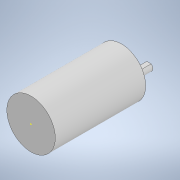
# Autodesk Inventor part: 29_Motore_6mm
Saved by Autodesk Inventor 2020.2 (Build 242310000, 310)
## iProperties
Created: 2020-01-17
Part Number: 29_Motore_6mm
Material: Generico
Document SubType Name: Modeling
Designer: socci
Density: 1 g/cm^3
Appearance: Default
Author: socci
Autodesk Inventor part; units mm, degrees
ref_plane "YZ Plane" through (0, 0, 0) normal (1, 0, 0) x (0, 1, 0)
ref_plane "XZ Plane" through (0, 0, 0) normal (0, 1, 0) x (-1, 0, 0)
ref_plane "XY Plane" through (0, 0, 0) normal (0, 0, 1) x (1, 0, 0)
sketch "Schizzo1" plane through (0, 0, 0) normal (0, 0, 1) x (1, 0, 0)
  circle A0 centre (0, 0) radius 18.5
  dimension "d0" = 37
  constraints: 1 centre point, 1 coincident
  measures "d0" diameter of A0
extrude "Estrusione1" add sketch "Schizzo1" along normal blind 69
sketch "Schizzo2" plane through (0, 0, 0) normal (0, 0, -1) x (-1, 0, 0)
  line L0 (0, 0) -> (15.3, 0)
  line L1 (0, 0) -> (15.3, 0) construction
  point P0 (7.65, 13.2502)
  point P1 (-7.65, 13.2502)
  point P2 (-15.3, 0)
  point P3 (-7.65, -13.2502)
  point P4 (7.65, -13.2502)
  dimension "d3" = 15.3
  dimension "d4" = 0
  dimension "d7" = 360
  constraints: 4 end point, 2 horizontal, 1 coincident, 1 collinear, 7 other
  measures "d3" distance of L0.start L0.end
  measures "d4" distance between parallel lines of L0 L1
hole "Foro1" at (7.65, 13.2502, 0) at (-7.65, 13.2502, 0) at (15.3, 0, 0) at (7.65, -13.2502, 0) at (-7.65, -13.2502, 0) at (-15.3, 0, 0) direction (0, 0, 1) diameter 2.459 depth 9 tip angle 118 thread size "M3x0.5" class "6H" standard "ISO Metric profile"
sketch "Schizzo3" plane through (0, 0, 0) normal (0, 0, -1) x (-1, 0, 0)
  circle A0 centre (0, 0) radius 18.5 projected
  line L0 (0, 18.5) -> (0, -0.9)
  line L1 (0, -0.9) -> (0, -6.9)
  circle A1 centre (0, -6.9) radius 6
  dimension "d16" = 19.4
  dimension "d17" = 6
  dimension "d18" = 12
  constraints: 4 end point, 1 centre point, 1 coincident, 1 point on line, 1 vertical, 1 vertical alignment, 1 other
  measures "d16" distance of L0.start L0.end
  measures "d17" distance of L0.end L1.end
  measures "d18" diameter of A1
extrude "Estrusione2" add sketch "Schizzo3" along normal blind 6 contours A1
sketch "Schizzo4" plane through (0, -6.9, -6) normal (0, 0, -1) x (-1, 0, 0)
  circle A0 centre (0, 0) radius 6 projected
  circle A1 centre (0, 0) radius 3
  point P0 (0, 6.9)
  dimension "d21" = 6
  constraints: 1 centre point, 1 coincident
  measures "d21" diameter of A1
extrude "Estrusione3" add sketch "Schizzo4" along normal blind 15 contours A1
sketch "Schizzo5" plane through (0, -6.9, -21) normal (0, 0, -1) x (-1, 0, 0)
  circle A0 centre (0, 0) radius 3
  circle A1 centre (0, 0) radius 3 projected
  line L0 (0, -3) -> (0, 2.5)
  line L1 (0, -3) -> (5.5, -3) construction
  line L2 (22.7528, -2.6034) -> (26.4877, -2.6034) construction
  line L3 (0, 2.5) -> (-1.6583, 2.5)
  line L4 (0, 2.5) -> (1.6583, 2.5)
  point P0 (0, 6.9)
  dimension "d24" = 6
  dimension "d25" = 5.5
  dimension "d26" = 90
  constraints: 10 end point, 4 horizontal, 3 point on circle, 1 centre point, 1 perpendicular, 1 vertical
  measures "d24" diameter of A0
  measures "d25" distance of L0.start L0.end
  measures "d26" angle of L1 L0
extrude "Estrusione4" cut sketch "Schizzo5" against normal blind 12 contours L4 L3 A0
sketch "Schizzo6" plane through (0, 0, 69) normal (0, 0, 1) x (1, 0, 0)
  point P0 (0, 0)
